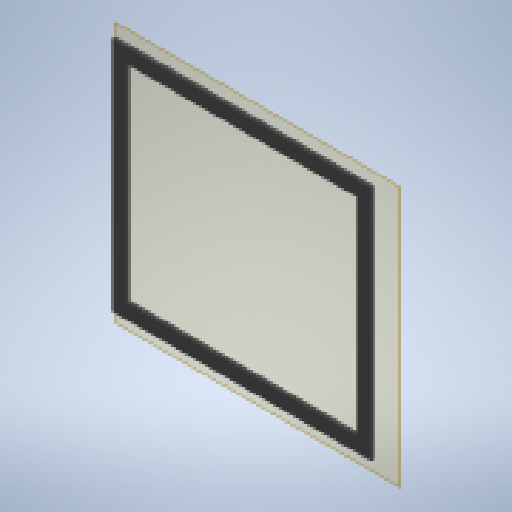
# Autodesk Inventor part: těsnění
Saved by Autodesk Inventor 2023 (Build 270158000, 158)
## iProperties
Created: 2023-04-04
Part Number: těsnění
Material: Rubber, Silicone
Document SubType Name: Modeling
Designer: lukyv
Mass: 9.93408 g
Surface Area: 99.3408 cm^2
Volume: 7.94726 cm^3
Density: 1.25 g/cm^3
Appearance: Rubber - Black
Author: lukyv
Autodesk Inventor part; units mm, degrees
ref_plane "YZ Plane" through (0, 0, 0) normal (1, 0, 0) x (0, 1, 0)
ref_plane "XZ Plane" through (0, 0, 0) normal (0, 1, 0) x (-1, 0, 0)
ref_plane "XY Plane" through (0, 0, 0) normal (0, 0, 1) x (1, 0, 0)
ref_plane "Work Plane1" through (6.7916, 0, 0) normal (0, 0, 1) x (1, 0, 0)
sketch "Sketch1" plane through (6.7916, 0, 0) normal (0, 0, 1) x (1, 0, 0)
  line L0 (54.3844, -55) -> (-67.9675, -55)
  line L1 (-67.9675, -55) -> (-67.9675, 55)
  line L2 (-67.9675, 55) -> (54.3844, 55)
  line L3 (54.3844, 55) -> (54.3844, -55)
  line L4 (-74.5533, -63) -> (60.9702, -63) projected
  line L5 (-75.9675, 61.5858) -> (-75.9675, -61.5858) projected
  line L6 (60.9702, 63) -> (-74.5533, 63) projected
  line L7 (62.3844, -61.5858) -> (62.3844, 61.5858) projected
  line L8 (-75.9675, 63) -> (62.3844, 63)
  line L9 (62.3844, 63) -> (62.3844, -63)
  line L10 (62.3844, -63) -> (-75.9675, -63)
  line L11 (-75.9675, -63) -> (-75.9675, 63)
  point P0 (-6.7916, 0)
  point P1 (-69.176, 61.5858)
  point P2 (-69.176, -61.5858)
  point P3 (-67.7617, -63)
  point P4 (67.7617, -63)
  point P5 (69.176, -61.5858)
  point P6 (69.176, 61.5858)
  point P7 (67.7617, 63)
  point P8 (-67.7617, 63)
  dimension "d0" = 8
  dimension "d1" = 8
  dimension "d2" = 8
  dimension "d3" = 8
  constraints: 16 end point, 4 parallel, 2 collinear, 2 horizontal, 2 perpendicular
  measures "d0" distance between parallel lines of L6 L2
  measures "d1" distance between parallel lines of L7 L3
  measures "d2" distance between parallel lines of L4 L0
  measures "d3" distance between parallel lines of L5 L1
extrude "Extrusion1" add sketch "Sketch1" along normal blind 2
equation "\"d1\" = d0"
equation "\"d2\" = d0"
equation "\"d3\" = d0"
body "Solid1"
